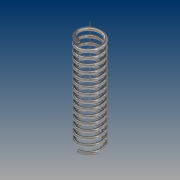
# Autodesk Inventor part: Lo_xo_phi_10x45
Saved by Autodesk Inventor 2021 (Build 250183000, 183)
## iProperties
Created: 2024-04-04
Part Number: Lo_xo_phi_10x45
Material: Steel, High Strength, Low Alloy
Document SubType Name: Modeling
Designer: Admin
Density: 7.85 g/cm^3
Appearance: Steel - Polished
Author: Admin
Autodesk Inventor part; units mm, degrees
ref_plane "YZ Plane" through (0, 0, 0) normal (1, 0, 0) x (0, 1, 0)
ref_plane "XZ Plane" through (0, 0, 0) normal (0, 1, 0) x (-1, 0, 0)
ref_plane "XY Plane" through (0, 0, 0) normal (0, 0, 1) x (1, 0, 0)
sketch "Sketch1" plane through (0, 0, 0) normal (1, 0, 0) x (0, 1, 0)
  circle A0 centre (0, 5.3) radius 0.68
  line L0 (0, 0) -> (5.4318, 0)
  dimension "d0" = 1.36
  dimension "d1" = 5.3
  constraints: 2 end point, 1 centre point, 1 horizontal
  measures "d0" diameter of A0
  measures "d1" distance of L0.start A0.centre
sketch "Sketch2" plane through (0, 0, 0) normal (0, 1, 0) x (-1, 0, 0)
  circle A0 centre (0, 0) radius 7.1863
  constraints: 1 centre point, 1 coincident
extrude "Extrusion1" add sketch "Sketch2" along normal blind 45
coil "Coil1" sketch "Sketch1" operation intersect axis through (0, 0, 0) along (0, 1, 0) pitch 3 turns 15 hand right
body "Solid1"
